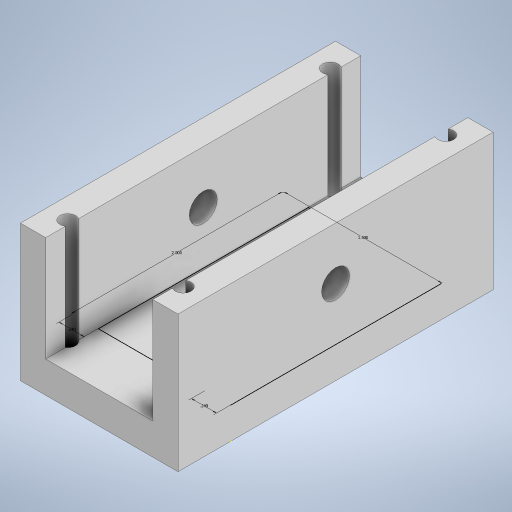
# Autodesk Inventor part: Sample Holder end for 8020-neutron-gen2-lid
Saved by Autodesk Inventor 2024.1 (Build 281209000, 209)
## iProperties
Created: 2022-02-14
Part Number: Sample Holder end for 8020-neutron-gen2-lid
Material: Generic
Document SubType Name: Modeling
Designer: Beaucage
Density: 1 g/cm^3
Appearance: Default
Author: Beaucage
Autodesk Inventor part; units mm, degrees
ref_plane "YZ Plane" through (0, 0, 0) normal (1, 0, 0) x (0, 1, 0)
ref_plane "XZ Plane" through (0, 0, 0) normal (0, 1, 0) x (-1, 0, 0)
ref_plane "XY Plane" through (0, 0, 0) normal (0, 0, 1) x (1, 0, 0)
sketch "Sketch1" plane through (0, 0, 0) normal (0, 1, 0) x (-1, 0, 0)
  line L0 (0, 0) -> (38.1, 0)
  line L1 (38.1, 0) -> (38.1, -50.8)
  line L2 (38.1, -50.8) -> (0, -50.8)
  line L3 (0, -50.8) -> (0, 0)
  line L4 (38.1, -50.8) -> (32.004, -50.8)
  line L5 (32.004, -50.8) -> (32.004, 0)
  line L6 (32.004, 0) -> (38.1, 0)
  line L7 (38.1, 0) -> (38.1, -50.8)
  line L8 (0, -50.8) -> (6.096, -50.8)
  line L9 (6.096, -50.8) -> (6.096, 0)
  line L10 (6.096, 0) -> (0, 0)
  line L11 (0, 0) -> (0, -50.8)
  dimension "d0" = 38.1
  dimension "d1" = 50.8
  dimension "d2" = 6.096
  dimension "d3" = 6.096
  constraints: 24 end point, 6 parallel, 3 horizontal, 3 perpendicular, 2 point on line
  measures "d0" distance of L1.end L2.end
  measures "d1" distance of L0.end L1.end
  measures "d2" distance of L5.end L6.end
  measures "d3" distance of L10.end L9.end
extrude "Extrusion1" add sketch "Sketch1" along normal blind 25.4 contours L0 L9 L2 L3 | L0 L1 L2 L5
extrude "Extrusion2" add sketch "Sketch1" against normal blind 5.08
sketch "Sketch2" plane through (0, 25.4, 0) normal (1, 0, 0) x (0, 0, -1)
  line L0 (50.8, 0) -> (0, 0) projected
  line L1 (25.4, 0) -> (25.4, -12.7)
  point P0 (0, -25.4)
  dimension "d8" = 12.7
  constraints: 2 end point, 1 midpoint, 1 vertical
  measures "d8" distance of L1.start L1.end
hole "Hole1" at (0, 12.7, -25.4) direction (-1, 0, 0) diameter 6.7564 end through all start extended yes clearance for "Socket Head Cap Screw" size "1/4" standard "Ansi Unified Screw Threads"
sketch "Sketch3" plane through (-6.096, 25.4, 0) normal (0, 0, 1) x (1, 0, 0)
  line L0 (6.096, -30.48) -> (6.096, 0) projected
  line L1 (0, 0) -> (6.096, 0) projected
  line L2 (0, -25.4) -> (0, 0) projected
  line L3 (-25.908, -25.4) -> (0, -25.4) projected
  line L4 (-25.908, -25.4) -> (-25.908, 0) projected
  line L5 (-32.004, 0) -> (-25.908, 0) projected
  line L6 (-32.004, -30.48) -> (-32.004, 0) projected
  line L7 (6.096, -30.48) -> (-32.004, -30.48) projected
  point P0 (6.096, -25.4)
extrude "Extrusion3" add sketch "Sketch3" along normal blind 12.7
sketch "Sketch4" plane through (0, 25.4, -50.8) normal (0, 0, -1) x (-1, 0, 0)
  line L0 (6.096, -25.4) -> (6.096, 0) projected
  line L1 (0, 0) -> (6.096, 0) projected
  line L2 (0, -30.48) -> (0, 0) projected
  line L3 (38.1, -30.48) -> (0, -30.48) projected
  line L4 (38.1, -30.48) -> (38.1, 0) projected
  line L5 (32.004, 0) -> (38.1, 0) projected
  line L6 (32.004, -25.4) -> (32.004, 0) projected
  line L7 (6.096, -25.4) -> (32.004, -25.4) projected
  point P0 (0, -25.4)
extrude "Extrusion4" add sketch "Sketch4" along normal blind 12.7
sketch "Sketch5" plane through (0, -5.08, 0) normal (0, -1, 0) x (1, 0, 0)
  line L0 (0, -63.5) -> (-38.1, -63.5) projected
  line L1 (-38.1, -63.5) -> (-38.1, 12.7) projected
  line L2 (0, 12.7) -> (0, -63.5) projected
  line L3 (-38.1, 12.7) -> (0, 12.7) projected
  line L4 (-26.67, -49.53) -> (-11.43, -49.53)
  line L5 (-11.43, -49.53) -> (-11.43, 1.27)
  line L6 (-11.43, 1.27) -> (-26.67, 1.27)
  line L7 (-26.67, 1.27) -> (-26.67, -49.53)
  line L8 (-26.67, -49.53) -> (-11.43, 1.27) construction
  line L9 (-11.43, -49.53) -> (-26.67, 1.27) construction
  line L10 (-19.05, 1.27) -> (-6.35, 1.27)
  line L11 (-6.35, 1.27) -> (-6.35, -43.18)
  line L12 (-6.35, -43.18) -> (-19.05, -43.18)
  line L13 (-19.05, -43.18) -> (-19.05, 1.27)
  line L14 (-19.05, 1.27) -> (-31.75, 1.27)
  line L15 (-31.75, 1.27) -> (-31.75, -43.18)
  line L16 (-31.75, -43.18) -> (-19.05, -43.18)
  line L17 (-19.05, -43.18) -> (-19.05, 1.27)
  point P0 (0, 0)
  point P1 (-19.05, -24.13)
  point P2 (-26.67, -43.18)
  point P3 (-11.43, 1.27)
  point P4 (-11.43, -43.18)
  dimension "d20" = 15.24
  dimension "d21" = 50.8
  dimension "d22" = 12.7
  dimension "d23" = 44.45
  dimension "d24" = 12.7
  constraints: 28 end point, 6 parallel, 3 horizontal, 3 midpoint, 3 perpendicular
  measures "d20" distance of L6.end L5.end
  measures "d21" distance of L5.end L4.end
  measures "d22" distance of L11.end L12.end
  measures "d23" distance of L10.end L11.end
  measures "d24" distance of L16.end L15.end
extrude "Extrusion5" add sketch "Sketch5" along normal blind 2.54
sketch "Sketch6" plane through (0, -7.62, 0) normal (0, -1, 0) x (1, 0, 0)
  point P0 (0, 0)
sketch "Sketch7" plane through (0, -7.62, 0) normal (0, -1, 0) x (1, 0, 0)
  line L0 (0, -63.5) -> (0, 12.7) projected
  line L1 (0, -63.5) -> (-5.08, -63.5)
  line L2 (-5.08, -63.5) -> (-5.08, -57.15)
  line L3 (-5.08, -57.15) -> (0, -57.15)
  line L4 (0, -57.15) -> (0, -63.5)
  line L5 (-38.1, 12.7) -> (-38.1, -63.5) projected
  line L6 (-38.1, -63.5) -> (-33.02, -63.5)
  line L7 (-33.02, -63.5) -> (-33.02, -57.15)
  line L8 (-33.02, -57.15) -> (-38.1, -57.15)
  line L9 (-38.1, -57.15) -> (-38.1, -63.5)
  line L10 (-38.1, 12.7) -> (-33.02, 12.7)
  line L11 (-33.02, 12.7) -> (-33.02, 6.35)
  line L12 (-33.02, 6.35) -> (-38.1, 6.35)
  line L13 (-38.1, 6.35) -> (-38.1, 12.7)
  line L14 (0, 12.7) -> (-5.08, 12.7)
  line L15 (-5.08, 12.7) -> (-5.08, 6.35)
  line L16 (-5.08, 6.35) -> (0, 6.35)
  line L17 (0, 6.35) -> (0, 12.7)
  point P0 (0, 0)
  dimension "d27" = 5.08
  dimension "d28" = 6.35
  dimension "d29" = 5.08
  dimension "d30" = 6.35
  dimension "d31" = 5.08
  dimension "d32" = 6.35
  dimension "d33" = 5.08
  constraints: 32 end point, 8 parallel, 4 horizontal, 4 perpendicular, 3 point on line
  measures "d27" distance of L2.end L3.end
  measures "d28" distance of L1.end L2.end
  measures "d29" distance of L8.end L7.end
  measures "d30" distance of L7.end L6.end
  measures "d31" distance of L11.end L12.end
  measures "d32" distance of L10.end L11.end
  measures "d33" distance of L16.end L15.end
hole "Hole2" at (-5.08, -7.62, -57.15) at (-33.02, -7.62, -57.15) at (-5.08, -7.62, 6.35) at (-33.02, -7.62, 6.35) direction (0, 1, 0) diameter 3.7973 end through all
body "Solid1"
